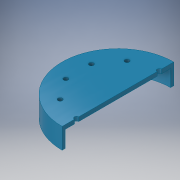
# Autodesk Inventor part: CoverPlateForWaterHalf
Saved by Autodesk Inventor 2018.2 (Build 222227000, 227)
## iProperties
Created: 2017-11-19
Part Number: CoverPlateForWaterHalf
Material: PET Plastic
Document SubType Name: Modeling
Designer: steele
Density: 1.541 g/cm^3
Appearance: Sky Blue Dark
Author: steele
Autodesk Inventor part; units mm, degrees
ref_plane "YZ Plane" through (0, 0, 0) normal (1, 0, 0) x (0, 1, 0)
ref_plane "XZ Plane" through (0, 0, 0) normal (0, 1, 0) x (-1, 0, 0)
ref_plane "XY Plane" through (0, 0, 0) normal (0, 0, 1) x (1, 0, 0)
sketch "Sketch1" plane through (0, 0, 0) normal (0, 1, 0) x (-1, 0, 0)
  circle A0 centre (0, 0) radius 85.725
  dimension "d0" = 171.45
  constraints: 1 centre point, 1 coincident
  measures "d0" diameter of A0
extrude "Extrusion1" add sketch "Sketch1" against normal blind 6.35
sketch "Sketch2" plane through (0, -6.35, 0) normal (0, -1, 0) x (1, 0, 0)
  circle A0 centre (0, 0) radius 85.725
  circle A1 centre (0, 0) radius 80.9625
  dimension "d3" = 161.925
  constraints: 2 centre point, 2 coincident
  measures "d3" diameter of A1
extrude "Extrusion2" add sketch "Sketch2" along normal blind 25.4
sketch "Sketch3" plane through (0, 0, 0) normal (0, 1, 0) x (1, 0, 0)
  arc A0 (0, -85.725) -> (0, 85.725) centre (0, 0) ccw
  circle A1 centre (0, 0) radius 85.725 projected
  line L0 (0, 85.725) -> (0, -85.725)
  constraints: 2 end point, 2 point on circle, 1 centre point, 1 coincident, 1 vertical, 1 vertical alignment, 1 other
extrude "Extrusion3" cut sketch "Sketch3" against normal through all contours L0 A0
sketch "Sketch4" plane through (0, 0, 0) normal (0, 1, 0) x (1, 0, 0)
  circle A0 centre (0, 0) radius 63.5 construction
  line L0 (0, 0) -> (-37.3244, -51.3726) construction
  line L1 (0, -85.725) -> (0, 85.725) construction
  point P0 (-60.3921, -19.6226)
  point P1 (-60.3921, 19.6226)
  point P2 (-37.3244, 51.3726)
  point P3 (0, 63.5)
  point P4 (37.3244, 51.3726)
  point P5 (60.3921, 19.6226)
  point P6 (60.3921, -19.6226)
  point P7 (37.3244, -51.3726)
  point P8 (0, -63.5)
  dimension "d8" = 127
  dimension "d9" = 36
  dimension "d12" = 360
  constraints: 2 coincident, 2 end point, 14 other
  measures "d9" angle of L0 L1
hole "Hole1" at (-37.3244, 0, 51.3726) at (-60.3921, 0, 19.6226) at (-60.3921, 0, -19.6226) at (-37.3244, 0, -51.3726) at (0, 0, -63.5) at (37.3244, 0, -51.3726) at (60.3921, 0, -19.6226) at (60.3921, 0, 19.6226) at (37.3244, 0, 51.3726) at (0, 0, 63.5) direction (0, -1, 0) diameter 6.7564 end through all clearance for "Flat Head Machine Screw (82)" size "1/4" standard "Ansi Unified Screw Threads"
body "Solid1"
